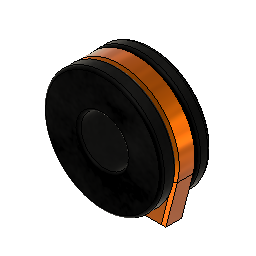
20021-014,015_vibration-damper (Autodesk Fusion 360 design; units mm, degrees)
Autodesk Fusion 360 part; units mm, degrees
sketch "Sketch1" plane through (0, 0, 0) normal (0, 1, 0) x (1, 0, 0)
  circle A0 centre (0, 0) radius 8.76
  arc A1 (-10.8907, 2.8205) -> (10.8907, 2.8205) centre (0, 0) ccw
  line L0 (-10.8907, 2.8205) -> (-8.705, 11.26)
  line L1 (10.8907, 2.8205) -> (8.705, 11.26)
  line L2 (8.705, 11.26) -> (-8.705, 11.26)
  point P0 (0, 8.76)
  dimension "d1" = 11.25
  dimension "d2" = 17.52
  dimension "d4" = 17.41
  dimension "d5" = 2.5
  constraint coincident A0.centre A1.centre
  constraint tangent A1 L0
  constraint tangent A1 L1
  constraint horizontal L2
  constraint horizontal A1.start A1.end
  constraint coincident A0 P0
  constraint vertical A0.centre P0
  measures "d1" radius of A1
  measures "d2" diameter of A0
  measures "d4" distance of L0.end L1.end
  measures "d5" distance of L2 P0
extrude "Extrude1" add sketch "Sketch1" along normal blind 4 makes body 1
chamfer "Chamfer1" distance 0.5 angle 45 10 edges at (-9.7978, 0, -7.0403) (0, 0, 11.25) (9.7978, 0, -7.0403) (-8.1672, 0, -3.1678) (-9.7978, 4, -7.0403) (0, 4, 11.25) (9.7978, 4, -7.0403) (-8.1672, 4, -3.1678) (0, 0, -11.26) (0, 4, -11.26) on bodies 1
sketch "Sketch2" plane through (0, 0, -11.26) normal (0, 0, -1) x (1, 0, 0)
  line L0 (-8.705, -3.5) -> (8.705, -3.5)
  line L1 (8.705, -3.5) -> (8.705, -0.5)
  line L2 (8.705, -0.5) -> (-8.705, -0.5)
  line L3 (-8.705, -0.5) -> (-8.705, -3.5)
  line L4 (-7, -2) -> (7, -2) construction
  point P0 (8.705, -2)
  point P1 (0, -2)
  dimension "d9" = 14
  constraint midpoint L1 P0
  constraint parallel L2 L4
  constraint coincident P0 L4
  constraint midpoint L4 P1
  constraint vertical origin P1
  measures "d9" distance of L4.start L4.end
hole "Hole1" at (-7, 2, -11.26) at (7, 2, -11.26) direction (0, 0, 1) diameter 2.076 depth 11.26 tip angle 118 bodies 1
thread "Thread1" "ISO Metric profile 2.5 M2.5x0.45 6H"
sketch "Sketch3" plane through (0, 0, 0) normal (1, 0, 0) x (0, 1, 0)
  line L0 (4, -9.26) -> (4, 9.26) construction
  line L1 (0, 9.26) -> (0, -9.26) construction
  line L2 (0, 0) -> (-2.85, 0) construction
  line L3 (-2.85, 0) -> (-2.85, 11.3)
  line L4 (-2.85, 11.3) -> (0, 11.3)
  line L5 (0, 11.3) -> (0, 8.3)
  line L6 (0, 8.3) -> (4, 8.3)
  line L7 (4, 8.3) -> (4, 11.3)
  line L8 (4, 11.3) -> (6.85, 11.3)
  line L9 (6.85, 11.3) -> (6.85, 0)
  line L10 (6.85, 0) -> (4, 0) construction
  line L11 (4, 0) -> (0, 0) construction
  line L12 (6.85, 4.55) -> (-2.85, 4.55)
  line L13 (2, 0) -> (2, 8.3) construction
  dimension "d13" = 8.3
  dimension "d14" = 11.3
  dimension "d15" = 9.7
  dimension "d16" = 4
  dimension "d17" = 4.55
  constraint coincident L2.start L11.end
  constraint perpendicular L1 L2
  constraint perpendicular L2 L3
  constraint perpendicular L3 L4
  constraint perpendicular L4 L5
  constraint perpendicular L0 L6
  constraint perpendicular L0 L8
  constraint perpendicular L8 L9
  constraint midpoint L0 L10.end
  constraint perpendicular L0 L10
  constraint coincident L9 L12.start
  constraint coincident L3 L12.end
  constraint perpendicular L3 L12
  constraint perpendicular L6 L7
  constraint coincident L4 L7.end
  constraint equal L4 L8
  constraint midpoint L11 L13.start
  constraint midpoint L6 L13.end
  constraint vertical L13
  measures "d13" distance of L6 L10
  measures "d14" distance of L8 L10
  measures "d15" distance of L3 L9
  measures "d16" distance of L5 L7
  measures "d17" distance of L10 L12
revolve "Revolve1" add sketch "Sketch3" angle 360 about axis through (0, 6.85, 0) along (0, -1, 0) separate body makes body 2
chamfer "Chamfer2" distance 0.75 angle 45 1 edges at (-10.5353, 6.85, 4.0863) on bodies 2
fillet "Fillet1" radius 0.5 9 faces at (0.9737, 0, 10.227) (0.9737, 4, 10.227) (1.1251, 5.4, 11.2438) (0.5241, 6.85, 8.5107) (0.5508, 6.35, 11.0363) (0.4137, 1.3333, 8.2897) (0.2268, 3.6167, 4.5443) (0.7874, -2.85, 8.991) (0.5633, -1.9, 11.286) on bodies 2
equation "d1 = ( 22.5 / 2 ) * 1 mm"
equation "d13 = ( 16.6 / 2 ) * 1 mm"
equation "d14 = ( 22.6 / 2 ) * 1 mm"
equation "d17 = ( 9.1 / 2 ) * 1 mm"
named bodies: "20021-014_vibration-damper-mount", "20021-015_vibration-damper-gasket"
